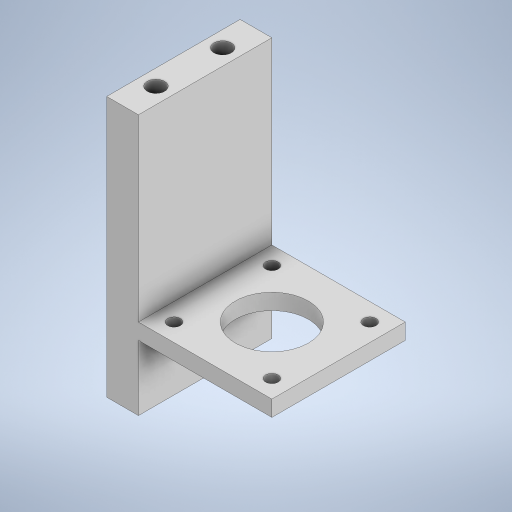
# Autodesk Inventor part: os2_polatforma
Saved by Autodesk Inventor 2024.3 (Build 283343000, 343)
## iProperties
Created: 2025-09-01
Part Number: os2_polatforma
Material: Ogólny
Document SubType Name: Modeling
Designer: User
Density: 1 g/cm^3
Appearance: Domyślna
Mass: 58.7306 g
Surface Area: 205.356 cm^2
Volume: 58.7306 cm^3
Author: User
Autodesk Inventor part; units mm, degrees
ref_plane "YZ Plane" through (0, 0, 0) normal (1, 0, 0) x (0, 1, 0)
ref_plane "XZ Plane" through (0, 0, 0) normal (0, 1, 0) x (-1, 0, 0)
ref_plane "XY Plane" through (0, 0, 0) normal (0, 0, 1) x (1, 0, 0)
sketch "Szkic1" plane through (0, 0, 0) normal (0, 1, 0) x (-1, 0, 0)
  line L0 (-3, 21) -> (3, 21)
  line L1 (3, 21) -> (3, -21)
  line L2 (3, -21) -> (-3, -21)
  line L3 (-3, -21) -> (-3, 21)
  line L4 (-3, 21) -> (3, -21) construction
  line L5 (3, 21) -> (-3, -21) construction
  line L6 (3, 21) -> (3, 0)
  line L7 (3, 0) -> (3, -21)
  line L8 (3, 10.5) -> (-3, 10.5)
  line L9 (3, -10.5) -> (-3, -10.5)
  line L10 (2, 21) -> (-8, 21)
  line L11 (-8, 21) -> (-8, -21)
  line L12 (-8, -21) -> (2, -21)
  line L13 (2, -21) -> (2, 21)
  line L14 (2, 21) -> (-8, -21) construction
  line L15 (-8, 21) -> (2, -21) construction
  circle A0 centre (-3, 10.5) radius 2.75
  circle A1 centre (-3, -10.5) radius 2.75
  point P0 (0, 0)
  point P1 (-3, 0)
  point P2 (-3, 21)
  point P3 (-3, -21)
  point P4 (3, -21)
  point P5 (-3, -21)
  point P6 (-3, 21)
  point P7 (3, 21)
  dimension "d0" = 6
  dimension "d1" = 42
  dimension "d2" = 6
  dimension "d3" = 6
  dimension "d4" = 10
  dimension "d5" = 5.5
  dimension "d6" = 5.5
  dimension "d29" = 42
  dimension "d30" = 21
  constraints: 32 end point, 8 midpoint, 4 parallel, 2 centre point, 2 coincident, 2 horizontal, 2 perpendicular, 2 point on line, 1 collinear
  measures "d0" distance of L1.end L2.end
  measures "d1" distance of L0.end L1.end
  measures "d2" distance of L8.start L8.end
  measures "d3" distance of L9.start L9.end
  measures "d4" distance of L12.end L11.end
  measures "d5" diameter of A0
  measures "d6" diameter of A1
  measures "d29" distance of L10.end L11.end
  measures "d30" distance of A1.centre A0.centre
extrude "Wyciągnięcie proste1" add sketch "Szkic1" along normal blind 82 contours L0 L13 L8 A0 L3 | L3 A0 A1 L12 L11 L10 | L13 L9 A1 L3 A0 L8 | L13 L2 L3 A1 L9
ref_plane "Płaszczyzna konstrukcyjna1" through (0, 20.5, 0) normal (0, -1, 0) x (1, 0, 0)
sketch "Szkic2" plane through (0, 20.5, 0) normal (0, -1, 0) x (1, 0, 0)
  line L0 (8, 21) -> (8, -21) projected
  line L1 (8, 0) -> (8, -21)
  line L2 (8, -21) -> (8, 21)
  line L3 (8, 21) -> (50, 21)
  line L4 (50, 21) -> (50, -21)
  line L5 (50, -21) -> (8, -21)
  line L6 (8, -21) -> (8, -15.4)
  line L7 (8, -15.4) -> (13.6, -15.4)
  circle A0 centre (13.6, -15.4) radius 2
  line L8 (8, 0) -> (50, 0)
  line L9 (29, 21) -> (29, -21)
  circle A1 centre (29, 0) radius 11.5
  circle A2 centre (44.4, -15.4) radius 2
  circle A3 centre (44.4, 15.4) radius 2
  circle A4 centre (13.6, 15.4) radius 2
  point P0 (0, 0)
  point P1 (9, 16)
  point P2 (9, -16)
  dimension "d10" = 21
  dimension "d11" = 42
  dimension "d12" = 42
  dimension "d13" = 5.6
  dimension "d14" = 5.6
  dimension "d15" = 4
  dimension "d16" = 23
  dimension "d19" = 360
  constraints: 18 end point, 5 centre point, 5 midpoint, 3 point on line, 2 parallel, 2 perpendicular, 1 coincident, 9 other
  measures "d10" distance of L1.start L1.end
  measures "d11" distance of L1.end L2.end
  measures "d12" distance of L2.end L3.end
  measures "d13" distance of L1.end L6.end
  measures "d14" distance of L6.end L7.end
  measures "d15" diameter of A0
  measures "d16" diameter of A1
extrude "Wyciągnięcie proste2" add sketch "Szkic2" against normal blind 3 contours L3 L9 A1 L8 L0 | L8 A1 L9 L5 L0 | L3 L4 L8 A1 L9 | A1 L8 L4 L5 L9
sketch "Szkic5" plane through (0, 20.5, 0) normal (0, -1, 0) x (1, 0, 0)
  circle A0 centre (13.6, 15.4) radius 2 projected
  circle A1 centre (13.6, 15.4) radius 2
  circle A2 centre (13.6, 15.4) radius 3
  circle A3 centre (29, 0) radius 11.5 projected
  circle A4 centre (29, 0) radius 11.5
  circle A5 centre (13.6, -15.4) radius 2
  circle A6 centre (13.6, -15.4) radius 3
  circle A7 centre (44.4, -15.4) radius 2
  circle A8 centre (44.4, -15.4) radius 3
  circle A9 centre (44.4, 15.4) radius 2
  circle A10 centre (44.4, 15.4) radius 3
  point P0 (0, 0)
  dimension "d40" = 6
  dimension "d43" = 360
  constraints: 9 centre point, 6 coincident, 17 other
  measures "d40" diameter of A2
extrude "Wyciągnięcie proste5" add sketch "Szkic5" along normal blind 3.5 contours A2 | A6 | A8 | A10
fillet "Zaokrąglenie3" radius 2 4 edges at (41.4, 20.5, -15.4) (41.4, 20.5, 15.4) (10.6, 20.5, 15.4) (10.6, 20.5, -15.4)
move faces "Przesuń1" translate (0, 2, 0) faces at (16.2182, 17, 15.0011) (16.2182, 17, -15.7989) (47.0182, 17, -15.7989) (47.0182, 17, 15.0011) (48.7236, 23.5, 4.8235)
